Autodesk Inventor part; units mm, degrees
(part 8 of 12)
  line L6268 (-29.2354, 17.1217) -> (-29.7413, 17.6276)
  line L6269 (-29.7413, 17.6276) -> (-30.4567, 17.6276)
  line L6270 (-30.4567, 17.6276) -> (-30.9626, 17.1217)
  line L6271 (-30.9626, 17.1217) -> (-30.9626, 16.4063)
  line L6272 (-30.9626, 16.4063) -> (-30.4567, 15.9004)
  line L6273 (-30.4567, 15.9004) -> (-29.7413, 15.9004)
  line L6274 (-29.7413, 15.9004) -> (-29.2354, 16.4063)
  circle A475 centre (-30.099, 16.764) radius 0.8636
  circle A476 centre (-30.099, 16.764) radius 0.8636
  line L6275 (-29.2354, 16.4063) -> (-29.2354, 17.1217)
  line L6276 (-29.2354, 17.1217) -> (-29.7413, 17.6276)
  line L6277 (-29.7413, 17.6276) -> (-30.4567, 17.6276)
  line L6278 (-30.4567, 17.6276) -> (-30.9626, 17.1217)
  line L6279 (-30.9626, 17.1217) -> (-30.9626, 16.4063)
  line L6280 (-30.9626, 16.4063) -> (-30.4567, 15.9004)
  line L6281 (-30.4567, 15.9004) -> (-29.7413, 15.9004)
  line L6282 (-29.7413, 15.9004) -> (-29.2354, 16.4063)
  line L6283 (-29.2354, 13.8663) -> (-29.2354, 14.5817)
  line L6284 (-29.2354, 14.5817) -> (-29.7413, 15.0876)
  line L6285 (-29.7413, 15.0876) -> (-30.4567, 15.0876)
  line L6286 (-30.4567, 15.0876) -> (-30.9626, 14.5817)
  line L6287 (-30.9626, 14.5817) -> (-30.9626, 13.8663)
  line L6288 (-30.9626, 13.8663) -> (-30.4567, 13.3604)
  line L6289 (-30.4567, 13.3604) -> (-29.7413, 13.3604)
  line L6290 (-29.7413, 13.3604) -> (-29.2354, 13.8663)
  circle A477 centre (-30.099, 14.224) radius 0.8636
  circle A478 centre (-30.099, 14.224) radius 0.8636
  line L6291 (-29.2354, 13.8663) -> (-29.2354, 14.5817)
  line L6292 (-29.2354, 14.5817) -> (-29.7413, 15.0876)
  line L6293 (-29.7413, 15.0876) -> (-30.4567, 15.0876)
  line L6294 (-30.4567, 15.0876) -> (-30.9626, 14.5817)
  line L6295 (-30.9626, 14.5817) -> (-30.9626, 13.8663)
  line L6296 (-30.9626, 13.8663) -> (-30.4567, 13.3604)
  line L6297 (-30.4567, 13.3604) -> (-29.7413, 13.3604)
  line L6298 (-29.7413, 13.3604) -> (-29.2354, 13.8663)
  line L6299 (-29.2354, 11.3263) -> (-29.2354, 12.0417)
  line L6300 (-29.2354, 12.0417) -> (-29.7413, 12.5476)
  line L6301 (-29.7413, 12.5476) -> (-30.4567, 12.5476)
  line L6302 (-30.4567, 12.5476) -> (-30.9626, 12.0417)
  line L6303 (-30.9626, 12.0417) -> (-30.9626, 11.3263)
  line L6304 (-30.9626, 11.3263) -> (-30.4567, 10.8204)
  line L6305 (-30.4567, 10.8204) -> (-29.7413, 10.8204)
  line L6306 (-29.7413, 10.8204) -> (-29.2354, 11.3263)
  circle A479 centre (-30.099, 11.684) radius 0.8636
  circle A480 centre (-30.099, 11.684) radius 0.8636
  line L6307 (-29.2354, 11.3263) -> (-29.2354, 12.0417)
  line L6308 (-29.2354, 12.0417) -> (-29.7413, 12.5476)
  line L6309 (-29.7413, 12.5476) -> (-30.4567, 12.5476)
  line L6310 (-30.4567, 12.5476) -> (-30.9626, 12.0417)
  line L6311 (-30.9626, 12.0417) -> (-30.9626, 11.3263)
  line L6312 (-30.9626, 11.3263) -> (-30.4567, 10.8204)
  line L6313 (-30.4567, 10.8204) -> (-29.7413, 10.8204)
  line L6314 (-29.7413, 10.8204) -> (-29.2354, 11.3263)
  line L6315 (-29.2354, 8.7863) -> (-29.2354, 9.5017)
  line L6316 (-29.2354, 9.5017) -> (-29.7413, 10.0076)
  line L6317 (-29.7413, 10.0076) -> (-30.4567, 10.0076)
  line L6318 (-30.4567, 10.0076) -> (-30.9626, 9.5017)
  line L6319 (-30.9626, 9.5017) -> (-30.9626, 8.7863)
  line L6320 (-30.9626, 8.7863) -> (-30.4567, 8.2804)
  line L6321 (-30.4567, 8.2804) -> (-29.7413, 8.2804)
  line L6322 (-29.7413, 8.2804) -> (-29.2354, 8.7863)
  circle A481 centre (-30.099, 9.144) radius 0.8636
  circle A482 centre (-30.099, 9.144) radius 0.8636
  line L6323 (-29.2354, 8.7863) -> (-29.2354, 9.5017)
  line L6324 (-29.2354, 9.5017) -> (-29.7413, 10.0076)
  line L6325 (-29.7413, 10.0076) -> (-30.4567, 10.0076)
  line L6326 (-30.4567, 10.0076) -> (-30.9626, 9.5017)
  line L6327 (-30.9626, 9.5017) -> (-30.9626, 8.7863)
  line L6328 (-30.9626, 8.7863) -> (-30.4567, 8.2804)
  line L6329 (-30.4567, 8.2804) -> (-29.7413, 8.2804)
  line L6330 (-29.7413, 8.2804) -> (-29.2354, 8.7863)
  line L6331 (-29.2354, 6.2463) -> (-29.2354, 6.9617)
  line L6332 (-29.2354, 6.9617) -> (-29.7413, 7.4676)
  line L6333 (-29.7413, 7.4676) -> (-30.4567, 7.4676)
  line L6334 (-30.4567, 7.4676) -> (-30.9626, 6.9617)
  line L6335 (-30.9626, 6.9617) -> (-30.9626, 6.2463)
  line L6336 (-30.9626, 6.2463) -> (-30.4567, 5.7404)
  line L6337 (-30.4567, 5.7404) -> (-29.7413, 5.7404)
  line L6338 (-29.7413, 5.7404) -> (-29.2354, 6.2463)
  circle A483 centre (-30.099, 6.604) radius 0.8636
  circle A484 centre (-30.099, 6.604) radius 0.8636
  line L6339 (-29.2354, 6.2463) -> (-29.2354, 6.9617)
  line L6340 (-29.2354, 6.9617) -> (-29.7413, 7.4676)
  line L6341 (-29.7413, 7.4676) -> (-30.4567, 7.4676)
  line L6342 (-30.4567, 7.4676) -> (-30.9626, 6.9617)
  line L6343 (-30.9626, 6.9617) -> (-30.9626, 6.2463)
  line L6344 (-30.9626, 6.2463) -> (-30.4567, 5.7404)
  line L6345 (-30.4567, 5.7404) -> (-29.7413, 5.7404)
  line L6346 (-29.7413, 5.7404) -> (-29.2354, 6.2463)
  line L6347 (-4.453, 11.714) -> (-4.453, 10.714)
  line L6348 (-4.453, 10.714) -> (-5.453, 10.714)
  line L6349 (-5.453, 10.714) -> (-5.453, 11.714)
  line L6350 (-5.453, 11.714) -> (-4.453, 11.714)
  line L6351 (-4.453, 10.114) -> (-4.453, 9.114)
  line L6352 (-4.453, 9.114) -> (-5.453, 9.114)
  line L6353 (-5.453, 9.114) -> (-5.453, 10.114)
  line L6354 (-5.453, 10.114) -> (-4.453, 10.114)
  line L6355 (-24.287, 6.977) -> (-23.287, 6.977)
  line L6356 (-23.287, 6.977) -> (-23.287, 5.977)
  line L6357 (-23.287, 5.977) -> (-24.287, 5.977)
  line L6358 (-24.287, 5.977) -> (-24.287, 6.977)
  line L6359 (-22.687, 6.977) -> (-21.687, 6.977)
  line L6360 (-21.687, 6.977) -> (-21.687, 5.977)
  line L6361 (-21.687, 5.977) -> (-22.687, 5.977)
  line L6362 (-22.687, 5.977) -> (-22.687, 6.977)
  line L6363 (-2.74, 31.099) -> (-3.74, 31.099)
  line L6364 (-3.74, 31.099) -> (-3.74, 32.099)
  line L6365 (-3.74, 32.099) -> (-2.74, 32.099)
  line L6366 (-2.74, 32.099) -> (-2.74, 31.099)
  line L6367 (-2.74, 28.099) -> (-3.74, 28.099)
  line L6368 (-3.74, 28.099) -> (-3.74, 29.099)
  line L6369 (-3.74, 29.099) -> (-2.74, 29.099)
  line L6370 (-2.74, 29.099) -> (-2.74, 28.099)
  line L6371 (-1.34, 28.099) -> (-2.34, 28.099)
  line L6372 (-2.34, 28.099) -> (-2.34, 29.099)
  line L6373 (-2.34, 29.099) -> (-1.34, 29.099)
  line L6374 (-1.34, 29.099) -> (-1.34, 28.099)
  line L6375 (-1.34, 31.099) -> (-2.34, 31.099)
  line L6376 (-2.34, 31.099) -> (-2.34, 32.099)
  line L6377 (-2.34, 32.099) -> (-1.34, 32.099)
  line L6378 (-1.34, 32.099) -> (-1.34, 31.099)
  line L6379 (-34.8585, 34.5556) -> (-34.1514, 35.2627)
  line L6380 (-34.1514, 35.2627) -> (-33.4443, 34.5556)
  line L6381 (-33.4443, 34.5556) -> (-34.1514, 33.8485)
  line L6382 (-34.1514, 33.8485) -> (-34.8585, 34.5556)
  line L6383 (-32.5957, 36.8184) -> (-31.8886, 37.5255)
  line L6384 (-31.8886, 37.5255) -> (-31.1815, 36.8184)
  line L6385 (-31.1815, 36.8184) -> (-31.8886, 36.1113)
  line L6386 (-31.8886, 36.1113) -> (-32.5957, 36.8184)
  line L6387 (-3.6714, 37.5255) -> (-2.9643, 36.8184)
  line L6388 (-2.9643, 36.8184) -> (-3.6714, 36.1113)
  line L6389 (-3.6714, 36.1113) -> (-4.3785, 36.8184)
  line L6390 (-4.3785, 36.8184) -> (-3.6714, 37.5255)
  line L6391 (-1.4086, 35.2627) -> (-0.7015, 34.5556)
  line L6392 (-0.7015, 34.5556) -> (-1.4086, 33.8485)
  line L6393 (-1.4086, 33.8485) -> (-2.1157, 34.5556)
  line L6394 (-2.1157, 34.5556) -> (-1.4086, 35.2627)
  circle A485 centre (-7.78, 36.068) radius 2.2225
  circle A486 centre (-7.78, 36.068) radius 1.778
  circle A487 centre (-7.78, 36.068) radius 1.778
  circle A488 centre (-7.78, 36.068) radius 2.2225
  circle A489 centre (-27.78, 36.068) radius 2.2225
  circle A490 centre (-27.78, 36.068) radius 1.778
  circle A491 centre (-27.78, 36.068) radius 1.778
  circle A492 centre (-27.78, 36.068) radius 2.2225
  line L6395 (-2.106, 23.519) -> (-3.106, 23.519)
  line L6396 (-3.106, 23.519) -> (-3.106, 24.519)
  line L6397 (-3.106, 24.519) -> (-2.106, 24.519)
  line L6398 (-2.106, 24.519) -> (-2.106, 23.519)
  line L6399 (-4.006, 23.519) -> (-5.006, 23.519)
  line L6400 (-5.006, 23.519) -> (-5.006, 24.519)
  line L6401 (-5.006, 24.519) -> (-4.006, 24.519)
  line L6402 (-4.006, 24.519) -> (-4.006, 23.519)
  line L6403 (-3.056, 25.619) -> (-4.056, 25.619)
  line L6404 (-4.056, 25.619) -> (-4.056, 26.619)
  line L6405 (-4.056, 26.619) -> (-3.056, 26.619)
  line L6406 (-3.056, 26.619) -> (-3.056, 25.619)
  line L6407 (-5.469, 25.519) -> (-5.469, 24.519)
  line L6408 (-5.469, 24.519) -> (-6.469, 24.519)
  line L6409 (-6.469, 24.519) -> (-6.469, 25.519)
  line L6410 (-6.469, 25.519) -> (-5.469, 25.519)
  line L6411 (-5.469, 26.369) -> (-5.469, 25.369)
  line L6412 (-5.469, 25.369) -> (-6.469, 25.369)
  line L6413 (-6.469, 25.369) -> (-6.469, 26.369)
  line L6414 (-6.469, 26.369) -> (-5.469, 26.369)
  line L6415 (-5.469, 24.669) -> (-5.469, 23.669)
  line L6416 (-5.469, 23.669) -> (-6.469, 23.669)
  line L6417 (-6.469, 23.669) -> (-6.469, 24.669)
  line L6418 (-6.469, 24.669) -> (-5.469, 24.669)
  line L6419 (-0.643, 25.519) -> (-0.643, 24.519)
  line L6420 (-0.643, 24.519) -> (-1.643, 24.519)
  line L6421 (-1.643, 24.519) -> (-1.643, 25.519)
  line L6422 (-1.643, 25.519) -> (-0.643, 25.519)
  line L6423 (-0.643, 26.369) -> (-0.643, 25.369)
  line L6424 (-0.643, 25.369) -> (-1.643, 25.369)
  line L6425 (-1.643, 25.369) -> (-1.643, 26.369)
  line L6426 (-1.643, 26.369) -> (-0.643, 26.369)
  line L6427 (-0.643, 24.669) -> (-0.643, 23.669)
  line L6428 (-0.643, 23.669) -> (-1.643, 23.669)
  line L6429 (-1.643, 23.669) -> (-1.643, 24.669)
  line L6430 (-1.643, 24.669) -> (-0.643, 24.669)
  line L6431 (-19.804, 30.599) -> (-18.804, 30.599)
  line L6432 (-18.804, 30.599) -> (-18.804, 29.599)
  line L6433 (-18.804, 29.599) -> (-19.804, 29.599)
  line L6434 (-19.804, 29.599) -> (-19.804, 30.599)
  line L6435 (-20.654, 30.599) -> (-19.654, 30.599)
  line L6436 (-19.654, 30.599) -> (-19.654, 29.599)
  line L6437 (-19.654, 29.599) -> (-20.654, 29.599)
  line L6438 (-20.654, 29.599) -> (-20.654, 30.599)
  line L6439 (-18.954, 30.599) -> (-17.954, 30.599)
  line L6440 (-17.954, 30.599) -> (-17.954, 29.599)
  line L6441 (-17.954, 29.599) -> (-18.954, 29.599)
  line L6442 (-18.954, 29.599) -> (-18.954, 30.599)
  line L6443 (-23.2, 32.7) -> (-23.2, 31.7)
  line L6444 (-23.2, 31.7) -> (-24.2, 31.7)
  line L6445 (-24.2, 31.7) -> (-24.2, 32.7)
  line L6446 (-24.2, 32.7) -> (-23.2, 32.7)
  line L6447 (-23.2, 33.55) -> (-23.2, 32.55)
  line L6448 (-23.2, 32.55) -> (-24.2, 32.55)
  line L6449 (-24.2, 32.55) -> (-24.2, 33.55)
  line L6450 (-24.2, 33.55) -> (-23.2, 33.55)
  line L6451 (-23.2, 31.85) -> (-23.2, 30.85)
  line L6452 (-23.2, 30.85) -> (-24.2, 30.85)
  line L6453 (-24.2, 30.85) -> (-24.2, 31.85)
  line L6454 (-24.2, 31.85) -> (-23.2, 31.85)
  line L6455 (-5.1385, 32.053) -> (-5.1385, 31.053)
  line L6456 (-5.1385, 31.053) -> (-6.1385, 31.053)
  line L6457 (-6.1385, 31.053) -> (-6.1385, 32.053)
  line L6458 (-6.1385, 32.053) -> (-5.1385, 32.053)
  line L6459 (-5.1385, 31.253) -> (-5.1385, 30.253)
  line L6460 (-5.1385, 30.253) -> (-6.1385, 30.253)
  line L6461 (-6.1385, 30.253) -> (-6.1385, 31.253)
  line L6462 (-6.1385, 31.253) -> (-5.1385, 31.253)
  line L6463 (-5.1385, 30.453) -> (-5.1385, 29.453)
  line L6464 (-5.1385, 29.453) -> (-6.1385, 29.453)
  line L6465 (-6.1385, 29.453) -> (-6.1385, 30.453)
  line L6466 (-6.1385, 30.453) -> (-5.1385, 30.453)
  line L6467 (-5.1385, 29.653) -> (-5.1385, 28.653)
  line L6468 (-5.1385, 28.653) -> (-6.1385, 28.653)
  line L6469 (-6.1385, 28.653) -> (-6.1385, 29.653)
  line L6470 (-6.1385, 29.653) -> (-5.1385, 29.653)
  line L6471 (-7.6885, 28.653) -> (-7.6885, 29.653)
  line L6472 (-7.6885, 29.653) -> (-6.6885, 29.653)
  line L6473 (-6.6885, 29.653) -> (-6.6885, 28.653)
  line L6474 (-6.6885, 28.653) -> (-7.6885, 28.653)
  line L6475 (-7.6885, 29.453) -> (-7.6885, 30.453)
  line L6476 (-7.6885, 30.453) -> (-6.6885, 30.453)
  line L6477 (-6.6885, 30.453) -> (-6.6885, 29.453)
  line L6478 (-6.6885, 29.453) -> (-7.6885, 29.453)
  line L6479 (-7.6885, 30.253) -> (-7.6885, 31.253)
  line L6480 (-7.6885, 31.253) -> (-6.6885, 31.253)
  line L6481 (-6.6885, 31.253) -> (-6.6885, 30.253)
  line L6482 (-6.6885, 30.253) -> (-7.6885, 30.253)
  line L6483 (-7.6885, 31.053) -> (-7.6885, 32.053)
  line L6484 (-7.6885, 32.053) -> (-6.6885, 32.053)
  line L6485 (-6.6885, 32.053) -> (-6.6885, 31.053)
  line L6486 (-6.6885, 31.053) -> (-7.6885, 31.053)
  line L6487 (-26.792, 24.941) -> (-26.792, 23.941)
  line L6488 (-26.792, 23.941) -> (-27.792, 23.941)
  line L6489 (-27.792, 23.941) -> (-27.792, 24.941)
  line L6490 (-27.792, 24.941) -> (-26.792, 24.941)
  line L6491 (-26.792, 24.141) -> (-26.792, 23.141)
  line L6492 (-26.792, 23.141) -> (-27.792, 23.141)
  line L6493 (-27.792, 23.141) -> (-27.792, 24.141)
  line L6494 (-27.792, 24.141) -> (-26.792, 24.141)
  line L6495 (-26.792, 23.341) -> (-26.792, 22.341)
  line L6496 (-26.792, 22.341) -> (-27.792, 22.341)
  line L6497 (-27.792, 22.341) -> (-27.792, 23.341)
  line L6498 (-27.792, 23.341) -> (-26.792, 23.341)
  line L6499 (-26.792, 22.541) -> (-26.792, 21.541)
  line L6500 (-26.792, 21.541) -> (-27.792, 21.541)
  line L6501 (-27.792, 21.541) -> (-27.792, 22.541)
  line L6502 (-27.792, 22.541) -> (-26.792, 22.541)
  line L6503 (-29.342, 21.541) -> (-29.342, 22.541)
  line L6504 (-29.342, 22.541) -> (-28.342, 22.541)
  line L6505 (-28.342, 22.541) -> (-28.342, 21.541)
  line L6506 (-28.342, 21.541) -> (-29.342, 21.541)
  line L6507 (-29.342, 22.341) -> (-29.342, 23.341)
  line L6508 (-29.342, 23.341) -> (-28.342, 23.341)
  line L6509 (-28.342, 23.341) -> (-28.342, 22.341)
  line L6510 (-28.342, 22.341) -> (-29.342, 22.341)
  line L6511 (-29.342, 23.141) -> (-29.342, 24.141)
  line L6512 (-29.342, 24.141) -> (-28.342, 24.141)
  line L6513 (-28.342, 24.141) -> (-28.342, 23.141)
  line L6514 (-28.342, 23.141) -> (-29.342, 23.141)
  line L6515 (-29.342, 23.941) -> (-29.342, 24.941)
  line L6516 (-29.342, 24.941) -> (-28.342, 24.941)
  line L6517 (-28.342, 24.941) -> (-28.342, 23.941)
  line L6518 (-28.342, 23.941) -> (-29.342, 23.941)
  line L6519 (-26.792, 32.434) -> (-26.792, 31.434)
  line L6520 (-26.792, 31.434) -> (-27.792, 31.434)
  line L6521 (-27.792, 31.434) -> (-27.792, 32.434)
  line L6522 (-27.792, 32.434) -> (-26.792, 32.434)
  line L6523 (-26.792, 31.634) -> (-26.792, 30.634)
  line L6524 (-26.792, 30.634) -> (-27.792, 30.634)
  line L6525 (-27.792, 30.634) -> (-27.792, 31.634)
  line L6526 (-27.792, 31.634) -> (-26.792, 31.634)
  line L6527 (-26.792, 30.834) -> (-26.792, 29.834)
  line L6528 (-26.792, 29.834) -> (-27.792, 29.834)
  line L6529 (-27.792, 29.834) -> (-27.792, 30.834)
  line L6530 (-27.792, 30.834) -> (-26.792, 30.834)
  line L6531 (-26.792, 30.034) -> (-26.792, 29.034)
  line L6532 (-26.792, 29.034) -> (-27.792, 29.034)
  line L6533 (-27.792, 29.034) -> (-27.792, 30.034)
  line L6534 (-27.792, 30.034) -> (-26.792, 30.034)
  line L6535 (-29.342, 29.034) -> (-29.342, 30.034)
  line L6536 (-29.342, 30.034) -> (-28.342, 30.034)
  line L6537 (-28.342, 30.034) -> (-28.342, 29.034)
  line L6538 (-28.342, 29.034) -> (-29.342, 29.034)
  line L6539 (-29.342, 29.834) -> (-29.342, 30.834)
  line L6540 (-29.342, 30.834) -> (-28.342, 30.834)
  line L6541 (-28.342, 30.834) -> (-28.342, 29.834)
  line L6542 (-28.342, 29.834) -> (-29.342, 29.834)
  line L6543 (-29.342, 30.634) -> (-29.342, 31.634)
  line L6544 (-29.342, 31.634) -> (-28.342, 31.634)
  line L6545 (-28.342, 31.634) -> (-28.342, 30.634)
  line L6546 (-28.342, 30.634) -> (-29.342, 30.634)
  line L6547 (-29.342, 31.434) -> (-29.342, 32.434)
  line L6548 (-29.342, 32.434) -> (-28.342, 32.434)
  line L6549 (-28.342, 32.434) -> (-28.342, 31.434)
  line L6550 (-28.342, 31.434) -> (-29.342, 31.434)
  line L6551 (-13.7, 30.325) -> (-14.7, 30.325)
  line L6552 (-14.7, 30.325) -> (-14.7, 31.325)
  line L6553 (-14.7, 31.325) -> (-13.7, 31.325)
  line L6554 (-13.7, 31.325) -> (-13.7, 30.325)
  line L6555 (-14.5, 30.325) -> (-15.5, 30.325)
  line L6556 (-15.5, 30.325) -> (-15.5, 31.325)
  line L6557 (-15.5, 31.325) -> (-14.5, 31.325)
  line L6558 (-14.5, 31.325) -> (-14.5, 30.325)
  line L6559 (-15.5, 32.875) -> (-14.5, 32.875)
  line L6560 (-14.5, 32.875) -> (-14.5, 31.875)
  line L6561 (-14.5, 31.875) -> (-15.5, 31.875)
  line L6562 (-15.5, 31.875) -> (-15.5, 32.875)
  line L6563 (-14.7, 32.875) -> (-13.7, 32.875)
  line L6564 (-13.7, 32.875) -> (-13.7, 31.875)
  line L6565 (-13.7, 31.875) -> (-14.7, 31.875)
  line L6566 (-14.7, 31.875) -> (-14.7, 32.875)
  line L6567 (-13.7367, 24.3158) -> (-14.7367, 24.3158)
  line L6568 (-14.7367, 24.3158) -> (-14.7367, 25.3158)
  line L6569 (-14.7367, 25.3158) -> (-13.7367, 25.3158)
  line L6570 (-13.7367, 25.3158) -> (-13.7367, 24.3158)
  line L6571 (-15.4512, 24.3158) -> (-16.4512, 24.3158)
  line L6572 (-16.4512, 24.3158) -> (-16.4512, 25.3158)
  line L6573 (-16.4512, 25.3158) -> (-15.4512, 25.3158)
  line L6574 (-15.4512, 25.3158) -> (-15.4512, 24.3158)
  line L6575 (-13.7367, 24.3412) -> (-14.7367, 24.3412)
  line L6576 (-14.7367, 24.3412) -> (-14.7367, 25.3412)
  line L6577 (-14.7367, 25.3412) -> (-13.7367, 25.3412)
  line L6578 (-13.7367, 25.3412) -> (-13.7367, 24.3412)
  line L6579 (-15.4512, 24.3412) -> (-16.4512, 24.3412)
  line L6580 (-16.4512, 24.3412) -> (-16.4512, 25.3412)
  line L6581 (-16.4512, 25.3412) -> (-15.4512, 25.3412)
  line L6582 (-15.4512, 25.3412) -> (-15.4512, 24.3412)
  line L6583 (-13.7748, 24.3666) -> (-14.7748, 24.3666)
  line L6584 (-14.7748, 24.3666) -> (-14.7748, 25.3666)
  line L6585 (-14.7748, 25.3666) -> (-13.7748, 25.3666)
  line L6586 (-13.7748, 25.3666) -> (-13.7748, 24.3666)
  line L6587 (-15.4512, 24.3666) -> (-16.4512, 24.3666)
  line L6588 (-16.4512, 24.3666) -> (-16.4512, 25.3666)
  line L6589 (-16.4512, 25.3666) -> (-15.4512, 25.3666)
  line L6590 (-15.4512, 25.3666) -> (-15.4512, 24.3666)
  line L6591 (-13.8256, 24.392) -> (-14.8256, 24.392)
  line L6592 (-14.8256, 24.392) -> (-14.8256, 25.392)
  line L6593 (-14.8256, 25.392) -> (-13.8256, 25.392)
  line L6594 (-13.8256, 25.392) -> (-13.8256, 24.392)
  line L6595 (-15.4512, 24.392) -> (-16.4512, 24.392)
  line L6596 (-16.4512, 24.392) -> (-16.4512, 25.392)
  line L6597 (-16.4512, 25.392) -> (-15.4512, 25.392)
  line L6598 (-15.4512, 25.392) -> (-15.4512, 24.392)
  line L6599 (-13.7287, 24.9047) -> (-13.7541, 24.9047)
  line L6600 (-13.7541, 24.9047) -> (-13.7541, 24.9301)
  line L6601 (-13.7541, 24.9301) -> (-13.7287, 24.9301)
  line L6602 (-13.7287, 24.9301) -> (-13.7287, 24.9047)
  line L6603 (-13.851, 24.4174) -> (-14.851, 24.4174)
  line L6604 (-14.851, 24.4174) -> (-14.851, 25.4174)
  line L6605 (-14.851, 25.4174) -> (-13.851, 25.4174)
  line L6606 (-13.851, 25.4174) -> (-13.851, 24.4174)
  line L6607 (-15.4512, 24.4174) -> (-16.4512, 24.4174)
  line L6608 (-16.4512, 24.4174) -> (-16.4512, 25.4174)
  line L6609 (-16.4512, 25.4174) -> (-15.4512, 25.4174)
  line L6610 (-15.4512, 25.4174) -> (-15.4512, 24.4174)
  line L6611 (-13.216, 24.4428) -> (-14.216, 24.4428)
  line L6612 (-14.216, 24.4428) -> (-14.216, 25.4428)
  line L6613 (-14.216, 25.4428) -> (-13.216, 25.4428)
  line L6614 (-13.216, 25.4428) -> (-13.216, 24.4428)
  line L6615 (-13.8764, 24.4428) -> (-14.8764, 24.4428)
  line L6616 (-14.8764, 24.4428) -> (-14.8764, 25.4428)
  line L6617 (-14.8764, 25.4428) -> (-13.8764, 25.4428)
  line L6618 (-13.8764, 25.4428) -> (-13.8764, 24.4428)
  line L6619 (-15.4512, 24.4428) -> (-16.4512, 24.4428)
  line L6620 (-16.4512, 24.4428) -> (-16.4512, 25.4428)
  line L6621 (-16.4512, 25.4428) -> (-15.4512, 25.4428)
  line L6622 (-15.4512, 25.4428) -> (-15.4512, 24.4428)
  line L6623 (-13.1906, 24.4682) -> (-14.1906, 24.4682)
  line L6624 (-14.1906, 24.4682) -> (-14.1906, 25.4682)
  line L6625 (-14.1906, 25.4682) -> (-13.1906, 25.4682)
  line L6626 (-13.1906, 25.4682) -> (-13.1906, 24.4682)
  line L6627 (-13.9018, 24.4682) -> (-14.9018, 24.4682)
  line L6628 (-14.9018, 24.4682) -> (-14.9018, 25.4682)
  line L6629 (-14.9018, 25.4682) -> (-13.9018, 25.4682)
  line L6630 (-13.9018, 25.4682) -> (-13.9018, 24.4682)
  line L6631 (-15.4639, 24.4682) -> (-16.4639, 24.4682)
  line L6632 (-16.4639, 24.4682) -> (-16.4639, 25.4682)
  line L6633 (-16.4639, 25.4682) -> (-15.4639, 25.4682)
  line L6634 (-15.4639, 25.4682) -> (-15.4639, 24.4682)
  line L6635 (-13.1652, 24.4936) -> (-14.1652, 24.4936)
  line L6636 (-14.1652, 24.4936) -> (-14.1652, 25.4936)
  line L6637 (-14.1652, 25.4936) -> (-13.1652, 25.4936)
  line L6638 (-13.1652, 25.4936) -> (-13.1652, 24.4936)
  line L6639 (-13.9272, 24.4936) -> (-14.9272, 24.4936)
  line L6640 (-14.9272, 24.4936) -> (-14.9272, 25.4936)
  line L6641 (-14.9272, 25.4936) -> (-13.9272, 25.4936)
  line L6642 (-13.9272, 25.4936) -> (-13.9272, 24.4936)
  line L6643 (-15.4639, 24.4936) -> (-16.4639, 24.4936)
  line L6644 (-16.4639, 24.4936) -> (-16.4639, 25.4936)
  line L6645 (-16.4639, 25.4936) -> (-15.4639, 25.4936)
  line L6646 (-15.4639, 25.4936) -> (-15.4639, 24.4936)
  line L6647 (-13.1525, 24.519) -> (-14.1525, 24.519)
  line L6648 (-14.1525, 24.519) -> (-14.1525, 25.519)
  line L6649 (-14.1525, 25.519) -> (-13.1525, 25.519)
  line L6650 (-13.1525, 25.519) -> (-13.1525, 24.519)
  line L6651 (-13.9526, 24.519) -> (-14.9526, 24.519)
  line L6652 (-14.9526, 24.519) -> (-14.9526, 25.519)
  line L6653 (-14.9526, 25.519) -> (-13.9526, 25.519)
  line L6654 (-13.9526, 25.519) -> (-13.9526, 24.519)
  line L6655 (-15.4639, 24.519) -> (-16.4639, 24.519)
  line L6656 (-16.4639, 24.519) -> (-16.4639, 25.519)
  line L6657 (-16.4639, 25.519) -> (-15.4639, 25.519)
  line L6658 (-15.4639, 25.519) -> (-15.4639, 24.519)
  line L6659 (-13.1271, 24.5444) -> (-14.1271, 24.5444)
  line L6660 (-14.1271, 24.5444) -> (-14.1271, 25.5444)
  line L6661 (-14.1271, 25.5444) -> (-13.1271, 25.5444)
  line L6662 (-13.1271, 25.5444) -> (-13.1271, 24.5444)
  line L6663 (-13.9653, 24.5444) -> (-14.9653, 24.5444)
  line L6664 (-14.9653, 24.5444) -> (-14.9653, 25.5444)
  line L6665 (-14.9653, 25.5444) -> (-13.9653, 25.5444)
  line L6666 (-13.9653, 25.5444) -> (-13.9653, 24.5444)
  line L6667 (-15.4639, 24.5444) -> (-16.4639, 24.5444)
  line L6668 (-16.4639, 24.5444) -> (-16.4639, 25.5444)
  line L6669 (-16.4639, 25.5444) -> (-15.4639, 25.5444)
  line L6670 (-15.4639, 25.5444) -> (-15.4639, 24.5444)
  line L6671 (-13.1144, 24.5698) -> (-14.1144, 24.5698)
  line L6672 (-14.1144, 24.5698) -> (-14.1144, 25.5698)
  line L6673 (-14.1144, 25.5698) -> (-13.1144, 25.5698)
  line L6674 (-13.1144, 25.5698) -> (-13.1144, 24.5698)
  line L6675 (-13.9907, 24.5698) -> (-14.9907, 24.5698)
  line L6676 (-14.9907, 24.5698) -> (-14.9907, 25.5698)
  line L6677 (-14.9907, 25.5698) -> (-13.9907, 25.5698)
  line L6678 (-13.9907, 25.5698) -> (-13.9907, 24.5698)
  line L6679 (-15.4639, 24.5698) -> (-16.4639, 24.5698)
  line L6680 (-16.4639, 24.5698) -> (-16.4639, 25.5698)
  line L6681 (-16.4639, 25.5698) -> (-15.4639, 25.5698)
  line L6682 (-15.4639, 25.5698) -> (-15.4639, 24.5698)
  line L6683 (-13.1017, 24.5952) -> (-14.1017, 24.5952)
  line L6684 (-14.1017, 24.5952) -> (-14.1017, 25.5952)
  line L6685 (-14.1017, 25.5952) -> (-13.1017, 25.5952)
  line L6686 (-13.1017, 25.5952) -> (-13.1017, 24.5952)
  line L6687 (-14.0034, 24.5952) -> (-15.0034, 24.5952)
  line L6688 (-15.0034, 24.5952) -> (-15.0034, 25.5952)
  line L6689 (-15.0034, 25.5952) -> (-14.0034, 25.5952)
  line L6690 (-14.0034, 25.5952) -> (-14.0034, 24.5952)
  line L6691 (-15.4639, 24.5952) -> (-16.4639, 24.5952)
  line L6692 (-16.4639, 24.5952) -> (-16.4639, 25.5952)
  line L6693 (-16.4639, 25.5952) -> (-15.4639, 25.5952)
  line L6694 (-15.4639, 25.5952) -> (-15.4639, 24.5952)
  line L6695 (-13.0763, 24.6206) -> (-14.0763, 24.6206)
  line L6696 (-14.0763, 24.6206) -> (-14.0763, 25.6206)
  line L6697 (-14.0763, 25.6206) -> (-13.0763, 25.6206)
  line L6698 (-13.0763, 25.6206) -> (-13.0763, 24.6206)
  line L6699 (-13.978, 24.6206) -> (-14.978, 24.6206)
  line L6700 (-14.978, 24.6206) -> (-14.978, 25.6206)
  line L6701 (-14.978, 25.6206) -> (-13.978, 25.6206)
  line L6702 (-13.978, 25.6206) -> (-13.978, 24.6206)
  line L6703 (-15.4639, 24.6206) -> (-16.4639, 24.6206)
  line L6704 (-16.4639, 24.6206) -> (-16.4639, 25.6206)
  line L6705 (-16.4639, 25.6206) -> (-15.4639, 25.6206)
  line L6706 (-15.4639, 25.6206) -> (-15.4639, 24.6206)
  line L6707 (-13.0636, 24.646) -> (-14.0636, 24.646)
  line L6708 (-14.0636, 24.646) -> (-14.0636, 25.646)
  line L6709 (-14.0636, 25.646) -> (-13.0636, 25.646)
  line L6710 (-13.0636, 25.646) -> (-13.0636, 24.646)
  line L6711 (-13.9526, 24.646) -> (-14.9526, 24.646)
  line L6712 (-14.9526, 24.646) -> (-14.9526, 25.646)
  line L6713 (-14.9526, 25.646) -> (-13.9526, 25.646)
  line L6714 (-13.9526, 25.646) -> (-13.9526, 24.646)
  line L6715 (-15.4639, 24.646) -> (-16.4639, 24.646)
  line L6716 (-16.4639, 24.646) -> (-16.4639, 25.646)
  line L6717 (-16.4639, 25.646) -> (-15.4639, 25.646)
  line L6718 (-15.4639, 25.646) -> (-15.4639, 24.646)
  line L6719 (-13.0509, 24.6714) -> (-14.0509, 24.6714)
  line L6720 (-14.0509, 24.6714) -> (-14.0509, 25.6714)
  line L6721 (-14.0509, 25.6714) -> (-13.0509, 25.6714)
  line L6722 (-13.0509, 25.6714) -> (-13.0509, 24.6714)
  line L6723 (-13.9272, 24.6714) -> (-14.9272, 24.6714)
  line L6724 (-14.9272, 24.6714) -> (-14.9272, 25.6714)
  line L6725 (-14.9272, 25.6714) -> (-13.9272, 25.6714)
  line L6726 (-13.9272, 25.6714) -> (-13.9272, 24.6714)
  line L6727 (-15.4766, 24.6714) -> (-16.4766, 24.6714)
  line L6728 (-16.4766, 24.6714) -> (-16.4766, 25.6714)
  line L6729 (-16.4766, 25.6714) -> (-15.4766, 25.6714)
  line L6730 (-15.4766, 25.6714) -> (-15.4766, 24.6714)
  line L6731 (-13.0382, 24.6968) -> (-14.0382, 24.6968)
  line L6732 (-14.0382, 24.6968) -> (-14.0382, 25.6968)
  line L6733 (-14.0382, 25.6968) -> (-13.0382, 25.6968)
  line L6734 (-13.0382, 25.6968) -> (-13.0382, 24.6968)
  line L6735 (-13.9145, 24.6968) -> (-14.9145, 24.6968)
  line L6736 (-14.9145, 24.6968) -> (-14.9145, 25.6968)
  line L6737 (-14.9145, 25.6968) -> (-13.9145, 25.6968)
  line L6738 (-13.9145, 25.6968) -> (-13.9145, 24.6968)
  line L6739 (-15.4766, 24.6968) -> (-16.4766, 24.6968)
  line L6740 (-16.4766, 24.6968) -> (-16.4766, 25.6968)
  line L6741 (-16.4766, 25.6968) -> (-15.4766, 25.6968)
  line L6742 (-15.4766, 25.6968) -> (-15.4766, 24.6968)
  line L6743 (-13.0255, 24.7222) -> (-14.0255, 24.7222)
  line L6744 (-14.0255, 24.7222) -> (-14.0255, 25.7222)
  line L6745 (-14.0255, 25.7222) -> (-13.0255, 25.7222)
  line L6746 (-13.0255, 25.7222) -> (-13.0255, 24.7222)
  line L6747 (-13.8891, 24.7222) -> (-14.8891, 24.7222)
  line L6748 (-14.8891, 24.7222) -> (-14.8891, 25.7222)
  line L6749 (-14.8891, 25.7222) -> (-13.8891, 25.7222)
  line L6750 (-13.8891, 25.7222) -> (-13.8891, 24.7222)
  line L6751 (-15.4766, 24.7222) -> (-16.4766, 24.7222)
  line L6752 (-16.4766, 24.7222) -> (-16.4766, 25.7222)
  line L6753 (-16.4766, 25.7222) -> (-15.4766, 25.7222)
  line L6754 (-15.4766, 25.7222) -> (-15.4766, 24.7222)
  line L6755 (-13.0128, 24.7476) -> (-14.0128, 24.7476)
  line L6756 (-14.0128, 24.7476) -> (-14.0128, 25.7476)
  line L6757 (-14.0128, 25.7476) -> (-13.0128, 25.7476)
  line L6758 (-13.0128, 25.7476) -> (-13.0128, 24.7476)
  line L6759 (-13.8637, 24.7476) -> (-14.8637, 24.7476)
  line L6760 (-14.8637, 24.7476) -> (-14.8637, 25.7476)
  line L6761 (-14.8637, 25.7476) -> (-13.8637, 25.7476)
  line L6762 (-13.8637, 25.7476) -> (-13.8637, 24.7476)
  line L6763 (-14.6892, 24.7476) -> (-15.6892, 24.7476)
  line L6764 (-15.6892, 24.7476) -> (-15.6892, 25.7476)
  line L6765 (-15.6892, 25.7476) -> (-14.6892, 25.7476)
  line L6766 (-14.6892, 25.7476) -> (-14.6892, 24.7476)
  line L6767 (-15.4766, 24.7476) -> (-16.4766, 24.7476)
  line L6768 (-16.4766, 24.7476) -> (-16.4766, 25.7476)
  line L6769 (-16.4766, 25.7476) -> (-15.4766, 25.7476)
  line L6770 (-15.4766, 25.7476) -> (-15.4766, 24.7476)
  line L6771 (-15.9973, 24.7476) -> (-16.9973, 24.7476)
  line L6772 (-16.9973, 24.7476) -> (-16.9973, 25.7476)
  line L6773 (-16.9973, 25.7476) -> (-15.9973, 25.7476)
  line L6774 (-15.9973, 25.7476) -> (-15.9973, 24.7476)
  line L6775 (-17.1403, 24.7476) -> (-18.1403, 24.7476)
  line L6776 (-18.1403, 24.7476) -> (-18.1403, 25.7476)
  line L6777 (-18.1403, 25.7476) -> (-17.1403, 25.7476)
  line L6778 (-17.1403, 25.7476) -> (-17.1403, 24.7476)
  line L6779 (-13.0001, 24.773) -> (-14.0001, 24.773)
  line L6780 (-14.0001, 24.773) -> (-14.0001, 25.773)
  line L6781 (-14.0001, 25.773) -> (-13.0001, 25.773)
  line L6782 (-13.0001, 25.773) -> (-13.0001, 24.773)
  line L6783 (-13.8383, 24.773) -> (-14.8383, 24.773)
  line L6784 (-14.8383, 24.773) -> (-14.8383, 25.773)
  line L6785 (-14.8383, 25.773) -> (-13.8383, 25.773)
  line L6786 (-13.8383, 25.773) -> (-13.8383, 24.773)
  line L6787 (-14.6765, 24.773) -> (-15.6765, 24.773)
  line L6788 (-15.6765, 24.773) -> (-15.6765, 25.773)
  line L6789 (-15.6765, 25.773) -> (-14.6765, 25.773)
  line L6790 (-14.6765, 25.773) -> (-14.6765, 24.773)
  line L6791 (-15.4766, 24.773) -> (-16.4766, 24.773)
  line L6792 (-16.4766, 24.773) -> (-16.4766, 25.773)
  line L6793 (-16.4766, 25.773) -> (-15.4766, 25.773)
  line L6794 (-15.4766, 25.773) -> (-15.4766, 24.773)
  line L6795 (-15.9973, 24.773) -> (-16.9973, 24.773)
  line L6796 (-16.9973, 24.773) -> (-16.9973, 25.773)
  line L6797 (-16.9973, 25.773) -> (-15.9973, 25.773)
  line L6798 (-15.9973, 25.773) -> (-15.9973, 24.773)
  line L6799 (-17.153, 24.773) -> (-18.153, 24.773)
  line L6800 (-18.153, 24.773) -> (-18.153, 25.773)
  line L6801 (-18.153, 25.773) -> (-17.153, 25.773)
  line L6802 (-17.153, 25.773) -> (-17.153, 24.773)
  line L6803 (-17.915, 24.773) -> (-18.915, 24.773)
  line L6804 (-18.915, 24.773) -> (-18.915, 25.773)
  line L6805 (-18.915, 25.773) -> (-17.915, 25.773)
  line L6806 (-17.915, 25.773) -> (-17.915, 24.773)
  line L6807 (-18.677, 24.773) -> (-19.677, 24.773)
  line L6808 (-19.677, 24.773) -> (-19.677, 25.773)
  line L6809 (-19.677, 25.773) -> (-18.677, 25.773)
  line L6810 (-18.677, 25.773) -> (-18.677, 24.773)
  line L6811 (-19.2358, 24.773) -> (-20.2358, 24.773)
  line L6812 (-20.2358, 24.773) -> (-20.2358, 25.773)
  line L6813 (-20.2358, 25.773) -> (-19.2358, 25.773)
  line L6814 (-19.2358, 25.773) -> (-19.2358, 24.773)
  line L6815 (-19.8327, 24.773) -> (-20.8327, 24.773)
  line L6816 (-20.8327, 24.773) -> (-20.8327, 25.773)
  line L6817 (-20.8327, 25.773) -> (-19.8327, 25.773)
  line L6818 (-19.8327, 25.773) -> (-19.8327, 24.773)
  line L6819 (-20.4677, 24.773) -> (-21.4677, 24.773)
  line L6820 (-21.4677, 24.773) -> (-21.4677, 25.773)
  line L6821 (-21.4677, 25.773) -> (-20.4677, 25.773)
  line L6822 (-20.4677, 25.773) -> (-20.4677, 24.773)
  line L6823 (-21.471, 24.773) -> (-22.471, 24.773)
  line L6824 (-22.471, 24.773) -> (-22.471, 25.773)
  line L6825 (-22.471, 25.773) -> (-21.471, 25.773)
  line L6826 (-21.471, 25.773) -> (-21.471, 24.773)
  line L6827 (-12.9874, 24.7984) -> (-13.9874, 24.7984)
  line L6828 (-13.9874, 24.7984) -> (-13.9874, 25.7984)
  line L6829 (-13.9874, 25.7984) -> (-12.9874, 25.7984)
  line L6830 (-12.9874, 25.7984) -> (-12.9874, 24.7984)
  line L6831 (-13.8256, 24.7984) -> (-14.8256, 24.7984)
  line L6832 (-14.8256, 24.7984) -> (-14.8256, 25.7984)
  line L6833 (-14.8256, 25.7984) -> (-13.8256, 25.7984)
  line L6834 (-13.8256, 25.7984) -> (-13.8256, 24.7984)
  line L6835 (-14.6765, 24.7984) -> (-15.6765, 24.7984)
  line L6836 (-15.6765, 24.7984) -> (-15.6765, 25.7984)
  line L6837 (-15.6765, 25.7984) -> (-14.6765, 25.7984)
  line L6838 (-14.6765, 25.7984) -> (-14.6765, 24.7984)
  line L6839 (-15.4766, 24.7984) -> (-16.4766, 24.7984)
  line L6840 (-16.4766, 24.7984) -> (-16.4766, 25.7984)
  line L6841 (-16.4766, 25.7984) -> (-15.4766, 25.7984)
  line L6842 (-15.4766, 25.7984) -> (-15.4766, 24.7984)
  line L6843 (-15.9846, 24.7984) -> (-16.9846, 24.7984)
  line L6844 (-16.9846, 24.7984) -> (-16.9846, 25.7984)
  line L6845 (-16.9846, 25.7984) -> (-15.9846, 25.7984)
  line L6846 (-15.9846, 25.7984) -> (-15.9846, 24.7984)
  line L6847 (-17.1276, 24.7984) -> (-18.1276, 24.7984)
  line L6848 (-18.1276, 24.7984) -> (-18.1276, 25.7984)
  line L6849 (-18.1276, 25.7984) -> (-17.1276, 25.7984)
  line L6850 (-17.1276, 25.7984) -> (-17.1276, 24.7984)
  line L6851 (-17.915, 24.7984) -> (-18.915, 24.7984)
  line L6852 (-18.915, 24.7984) -> (-18.915, 25.7984)
  line L6853 (-18.915, 25.7984) -> (-17.915, 25.7984)
  line L6854 (-17.915, 25.7984) -> (-17.915, 24.7984)
  line L6855 (-18.677, 24.7984) -> (-19.677, 24.7984)
  line L6856 (-19.677, 24.7984) -> (-19.677, 25.7984)
  line L6857 (-19.677, 25.7984) -> (-18.677, 25.7984)
  line L6858 (-18.677, 25.7984) -> (-18.677, 24.7984)
  line L6859 (-19.2358, 24.7984) -> (-20.2358, 24.7984)
  line L6860 (-20.2358, 24.7984) -> (-20.2358, 25.7984)
  line L6861 (-20.2358, 25.7984) -> (-19.2358, 25.7984)
  line L6862 (-19.2358, 25.7984) -> (-19.2358, 24.7984)
  line L6863 (-19.8454, 24.7984) -> (-20.8454, 24.7984)
  line L6864 (-20.8454, 24.7984) -> (-20.8454, 25.7984)
  line L6865 (-20.8454, 25.7984) -> (-19.8454, 25.7984)
  line L6866 (-19.8454, 25.7984) -> (-19.8454, 24.7984)
  line L6867 (-20.4677, 24.7984) -> (-21.4677, 24.7984)
  line L6868 (-21.4677, 24.7984) -> (-21.4677, 25.7984)
  line L6869 (-21.4677, 25.7984) -> (-20.4677, 25.7984)
  line L6870 (-20.4677, 25.7984) -> (-20.4677, 24.7984)
  line L6871 (-21.471, 24.7984) -> (-22.471, 24.7984)
  line L6872 (-22.471, 24.7984) -> (-22.471, 25.7984)
  line L6873 (-22.471, 25.7984) -> (-21.471, 25.7984)
  line L6874 (-21.471, 25.7984) -> (-21.471, 24.7984)
  line L6875 (-12.9874, 24.8238) -> (-13.9874, 24.8238)
  line L6876 (-13.9874, 24.8238) -> (-13.9874, 25.8238)
  line L6877 (-13.9874, 25.8238) -> (-12.9874, 25.8238)
  line L6878 (-12.9874, 25.8238) -> (-12.9874, 24.8238)
  line L6879 (-13.8002, 24.8238) -> (-14.8002, 24.8238)
  line L6880 (-14.8002, 24.8238) -> (-14.8002, 25.8238)
  line L6881 (-14.8002, 25.8238) -> (-13.8002, 25.8238)
  line L6882 (-13.8002, 25.8238) -> (-13.8002, 24.8238)
  line L6883 (-14.6638, 24.8238) -> (-15.6638, 24.8238)
  line L6884 (-15.6638, 24.8238) -> (-15.6638, 25.8238)
  line L6885 (-15.6638, 25.8238) -> (-14.6638, 25.8238)
  line L6886 (-14.6638, 25.8238) -> (-14.6638, 24.8238)
  line L6887 (-15.4766, 24.8238) -> (-16.4766, 24.8238)
  line L6888 (-16.4766, 24.8238) -> (-16.4766, 25.8238)
  line L6889 (-16.4766, 25.8238) -> (-15.4766, 25.8238)
  line L6890 (-15.4766, 25.8238) -> (-15.4766, 24.8238)
  line L6891 (-15.9846, 24.8238) -> (-16.9846, 24.8238)
  line L6892 (-16.9846, 24.8238) -> (-16.9846, 25.8238)
  line L6893 (-16.9846, 25.8238) -> (-15.9846, 25.8238)
  line L6894 (-15.9846, 25.8238) -> (-15.9846, 24.8238)
  line L6895 (-17.1022, 24.8238) -> (-18.1022, 24.8238)
  line L6896 (-18.1022, 24.8238) -> (-18.1022, 25.8238)
  line L6897 (-18.1022, 25.8238) -> (-17.1022, 25.8238)
  line L6898 (-17.1022, 25.8238) -> (-17.1022, 24.8238)
  line L6899 (-17.915, 24.8238) -> (-18.915, 24.8238)
  line L6900 (-18.915, 24.8238) -> (-18.915, 25.8238)
  line L6901 (-18.915, 25.8238) -> (-17.915, 25.8238)
  line L6902 (-17.915, 25.8238) -> (-17.915, 24.8238)
  line L6903 (-18.677, 24.8238) -> (-19.677, 24.8238)
  line L6904 (-19.677, 24.8238) -> (-19.677, 25.8238)
  line L6905 (-19.677, 25.8238) -> (-18.677, 25.8238)
  line L6906 (-18.677, 25.8238) -> (-18.677, 24.8238)
  line L6907 (-19.2358, 24.8238) -> (-20.2358, 24.8238)
  line L6908 (-20.2358, 24.8238) -> (-20.2358, 25.8238)
  line L6909 (-20.2358, 25.8238) -> (-19.2358, 25.8238)
  line L6910 (-19.2358, 25.8238) -> (-19.2358, 24.8238)
  line L6911 (-19.8454, 24.8238) -> (-20.8454, 24.8238)
  line L6912 (-20.8454, 24.8238) -> (-20.8454, 25.8238)
  line L6913 (-20.8454, 25.8238) -> (-19.8454, 25.8238)
  line L6914 (-19.8454, 25.8238) -> (-19.8454, 24.8238)
  line L6915 (-20.4804, 24.8238) -> (-21.4804, 24.8238)
  line L6916 (-21.4804, 24.8238) -> (-21.4804, 25.8238)
  line L6917 (-21.4804, 25.8238) -> (-20.4804, 25.8238)
  line L6918 (-20.4804, 25.8238) -> (-20.4804, 24.8238)
  line L6919 (-21.471, 24.8238) -> (-22.471, 24.8238)
  line L6920 (-22.471, 24.8238) -> (-22.471, 25.8238)
  line L6921 (-22.471, 25.8238) -> (-21.471, 25.8238)
  line L6922 (-21.471, 25.8238) -> (-21.471, 24.8238)
  line L6923 (-12.9747, 24.8492) -> (-13.9747, 24.8492)
  line L6924 (-13.9747, 24.8492) -> (-13.9747, 25.8492)
  line L6925 (-13.9747, 25.8492) -> (-12.9747, 25.8492)
  line L6926 (-12.9747, 25.8492) -> (-12.9747, 24.8492)
  line L6927 (-13.7748, 24.8492) -> (-14.7748, 24.8492)
  line L6928 (-14.7748, 24.8492) -> (-14.7748, 25.8492)
  line L6929 (-14.7748, 25.8492) -> (-13.7748, 25.8492)
  line L6930 (-13.7748, 25.8492) -> (-13.7748, 24.8492)
  line L6931 (-14.6384, 24.8492) -> (-15.6384, 24.8492)
  line L6932 (-15.6384, 24.8492) -> (-15.6384, 25.8492)
  line L6933 (-15.6384, 25.8492) -> (-14.6384, 25.8492)
  line L6934 (-14.6384, 25.8492) -> (-14.6384, 24.8492)
  line L6935 (-15.7941, 24.8492) -> (-16.7941, 24.8492)
  line L6936 (-16.7941, 24.8492) -> (-16.7941, 25.8492)
  line L6937 (-16.7941, 25.8492) -> (-15.7941, 25.8492)
  line L6938 (-15.7941, 25.8492) -> (-15.7941, 24.8492)
  line L6939 (-17.1022, 24.8492) -> (-18.1022, 24.8492)
  line L6940 (-18.1022, 24.8492) -> (-18.1022, 25.8492)
  line L6941 (-18.1022, 25.8492) -> (-17.1022, 25.8492)
  line L6942 (-17.1022, 25.8492) -> (-17.1022, 24.8492)
  line L6943 (-17.9277, 24.8492) -> (-18.9277, 24.8492)
  line L6944 (-18.9277, 24.8492) -> (-18.9277, 25.8492)
  line L6945 (-18.9277, 25.8492) -> (-17.9277, 25.8492)
  line L6946 (-17.9277, 25.8492) -> (-17.9277, 24.8492)
  line L6947 (-18.677, 24.8492) -> (-19.677, 24.8492)
  line L6948 (-19.677, 24.8492) -> (-19.677, 25.8492)
  line L6949 (-19.677, 25.8492) -> (-18.677, 25.8492)
  line L6950 (-18.677, 25.8492) -> (-18.677, 24.8492)
  line L6951 (-19.2358, 24.8492) -> (-20.2358, 24.8492)
  line L6952 (-20.2358, 24.8492) -> (-20.2358, 25.8492)
  line L6953 (-20.2358, 25.8492) -> (-19.2358, 25.8492)
  line L6954 (-19.2358, 25.8492) -> (-19.2358, 24.8492)
  line L6955 (-19.8454, 24.8492) -> (-20.8454, 24.8492)
  line L6956 (-20.8454, 24.8492) -> (-20.8454, 25.8492)
  line L6957 (-20.8454, 25.8492) -> (-19.8454, 25.8492)
  line L6958 (-19.8454, 25.8492) -> (-19.8454, 24.8492)
  line L6959 (-20.4804, 24.8492) -> (-21.4804, 24.8492)
  line L6960 (-21.4804, 24.8492) -> (-21.4804, 25.8492)
  line L6961 (-21.4804, 25.8492) -> (-20.4804, 25.8492)
  line L6962 (-20.4804, 25.8492) -> (-20.4804, 24.8492)
  line L6963 (-21.471, 24.8492) -> (-22.471, 24.8492)
  line L6964 (-22.471, 24.8492) -> (-22.471, 25.8492)
  line L6965 (-22.471, 25.8492) -> (-21.471, 25.8492)
  line L6966 (-21.471, 25.8492) -> (-21.471, 24.8492)
  line L6967 (-12.962, 24.8746) -> (-13.962, 24.8746)
  line L6968 (-13.962, 24.8746) -> (-13.962, 25.8746)
  line L6969 (-13.962, 25.8746) -> (-12.962, 25.8746)
  line L6970 (-12.962, 25.8746) -> (-12.962, 24.8746)
  line L6971 (-13.7494, 24.8746) -> (-14.7494, 24.8746)
  line L6972 (-14.7494, 24.8746) -> (-14.7494, 25.8746)
  line L6973 (-14.7494, 25.8746) -> (-13.7494, 25.8746)
  line L6974 (-13.7494, 25.8746) -> (-13.7494, 24.8746)
  line L6975 (-14.6257, 24.8746) -> (-15.6257, 24.8746)
  line L6976 (-15.6257, 24.8746) -> (-15.6257, 25.8746)
  line L6977 (-15.6257, 25.8746) -> (-14.6257, 25.8746)
  line L6978 (-14.6257, 25.8746) -> (-14.6257, 24.8746)
  line L6979 (-15.8068, 24.8746) -> (-16.8068, 24.8746)
  line L6980 (-16.8068, 24.8746) -> (-16.8068, 25.8746)
  line L6981 (-16.8068, 25.8746) -> (-15.8068, 25.8746)
  line L6982 (-15.8068, 25.8746) -> (-15.8068, 24.8746)
  line L6983 (-17.0895, 24.8746) -> (-18.0895, 24.8746)
  line L6984 (-18.0895, 24.8746) -> (-18.0895, 25.8746)
  line L6985 (-18.0895, 25.8746) -> (-17.0895, 25.8746)
  line L6986 (-17.0895, 25.8746) -> (-17.0895, 24.8746)
  line L6987 (-17.9404, 24.8746) -> (-18.9404, 24.8746)
  line L6988 (-18.9404, 24.8746) -> (-18.9404, 25.8746)
  line L6989 (-18.9404, 25.8746) -> (-17.9404, 25.8746)
  line L6990 (-17.9404, 25.8746) -> (-17.9404, 24.8746)
  line L6991 (-18.677, 24.8746) -> (-19.677, 24.8746)
  line L6992 (-19.677, 24.8746) -> (-19.677, 25.8746)
  line L6993 (-19.677, 25.8746) -> (-18.677, 25.8746)
  line L6994 (-18.677, 25.8746) -> (-18.677, 24.8746)
  line L6995 (-19.2358, 24.8746) -> (-20.2358, 24.8746)
  line L6996 (-20.2358, 24.8746) -> (-20.2358, 25.8746)
  line L6997 (-20.2358, 25.8746) -> (-19.2358, 25.8746)
  line L6998 (-19.2358, 25.8746) -> (-19.2358, 24.8746)
  line L6999 (-19.8581, 24.8746) -> (-20.8581, 24.8746)
  line L7000 (-20.8581, 24.8746) -> (-20.8581, 25.8746)
  line L7001 (-20.8581, 25.8746) -> (-19.8581, 25.8746)
  line L7002 (-19.8581, 25.8746) -> (-19.8581, 24.8746)
  line L7003 (-20.4804, 24.8746) -> (-21.4804, 24.8746)
  line L7004 (-21.4804, 24.8746) -> (-21.4804, 25.8746)
  line L7005 (-21.4804, 25.8746) -> (-20.4804, 25.8746)
  line L7006 (-20.4804, 25.8746) -> (-20.4804, 24.8746)
  line L7007 (-21.4837, 24.8746) -> (-22.4837, 24.8746)
  line L7008 (-22.4837, 24.8746) -> (-22.4837, 25.8746)
  line L7009 (-22.4837, 25.8746) -> (-21.4837, 25.8746)
  line L7010 (-21.4837, 25.8746) -> (-21.4837, 24.8746)
  line L7011 (-12.9493, 24.9) -> (-13.9493, 24.9)
  line L7012 (-13.9493, 24.9) -> (-13.9493, 25.9)
  line L7013 (-13.9493, 25.9) -> (-12.9493, 25.9)
  line L7014 (-12.9493, 25.9) -> (-12.9493, 24.9)
  line L7015 (-13.7367, 24.9) -> (-14.7367, 24.9)
  line L7016 (-14.7367, 24.9) -> (-14.7367, 25.9)
  line L7017 (-14.7367, 25.9) -> (-13.7367, 25.9)
  line L7018 (-13.7367, 25.9) -> (-13.7367, 24.9)
  line L7019 (-14.6257, 24.9) -> (-15.6257, 24.9)
  line L7020 (-15.6257, 24.9) -> (-15.6257, 25.9)
  line L7021 (-15.6257, 25.9) -> (-14.6257, 25.9)
  line L7022 (-14.6257, 25.9) -> (-14.6257, 24.9)
  line L7023 (-15.8195, 24.9) -> (-16.8195, 24.9)
  line L7024 (-16.8195, 24.9) -> (-16.8195, 25.9)
  line L7025 (-16.8195, 25.9) -> (-15.8195, 25.9)
  line L7026 (-15.8195, 25.9) -> (-15.8195, 24.9)
  line L7027 (-17.0768, 24.9) -> (-18.0768, 24.9)
  line L7028 (-18.0768, 24.9) -> (-18.0768, 25.9)
  line L7029 (-18.0768, 25.9) -> (-17.0768, 25.9)
  line L7030 (-17.0768, 25.9) -> (-17.0768, 24.9)
  line L7031 (-17.9404, 24.9) -> (-18.9404, 24.9)
  line L7032 (-18.9404, 24.9) -> (-18.9404, 25.9)
  line L7033 (-18.9404, 25.9) -> (-17.9404, 25.9)
  line L7034 (-17.9404, 25.9) -> (-17.9404, 24.9)
  line L7035 (-18.677, 24.9) -> (-19.677, 24.9)
  line L7036 (-19.677, 24.9) -> (-19.677, 25.9)
  line L7037 (-19.677, 25.9) -> (-18.677, 25.9)
  line L7038 (-18.677, 25.9) -> (-18.677, 24.9)
  line L7039 (-19.2358, 24.9) -> (-20.2358, 24.9)
  line L7040 (-20.2358, 24.9) -> (-20.2358, 25.9)
  line L7041 (-20.2358, 25.9) -> (-19.2358, 25.9)
  line L7042 (-19.2358, 25.9) -> (-19.2358, 24.9)
  line L7043 (-19.8454, 24.9) -> (-20.8454, 24.9)
  line L7044 (-20.8454, 24.9) -> (-20.8454, 25.9)
  line L7045 (-20.8454, 25.9) -> (-19.8454, 25.9)
  line L7046 (-19.8454, 25.9) -> (-19.8454, 24.9)
  line L7047 (-20.4804, 24.9) -> (-21.4804, 24.9)
  line L7048 (-21.4804, 24.9) -> (-21.4804, 25.9)
  line L7049 (-21.4804, 25.9) -> (-20.4804, 25.9)
  line L7050 (-20.4804, 25.9) -> (-20.4804, 24.9)
  line L7051 (-21.471, 24.9) -> (-22.471, 24.9)
  line L7052 (-22.471, 24.9) -> (-22.471, 25.9)
  line L7053 (-22.471, 25.9) -> (-21.471, 25.9)
  line L7054 (-21.471, 25.9) -> (-21.471, 24.9)
  line L7055 (-12.9493, 24.9254) -> (-13.9493, 24.9254)
  line L7056 (-13.9493, 24.9254) -> (-13.9493, 25.9254)
  line L7057 (-13.9493, 25.9254) -> (-12.9493, 25.9254)
  line L7058 (-12.9493, 25.9254) -> (-12.9493, 24.9254)
  line L7059 (-13.7113, 24.9254) -> (-14.7113, 24.9254)
  line L7060 (-14.7113, 24.9254) -> (-14.7113, 25.9254)
  line L7061 (-14.7113, 25.9254) -> (-13.7113, 25.9254)
  line L7062 (-13.7113, 25.9254) -> (-13.7113, 24.9254)
  line L7063 (-14.6003, 24.9254) -> (-15.6003, 24.9254)
  line L7064 (-15.6003, 24.9254) -> (-15.6003, 25.9254)
  line L7065 (-15.6003, 25.9254) -> (-14.6003, 25.9254)
  line L7066 (-14.6003, 25.9254) -> (-14.6003, 24.9254)
  line L7067 (-15.8322, 24.9254) -> (-16.8322, 24.9254)
  line L7068 (-16.8322, 24.9254) -> (-16.8322, 25.9254)
  line L7069 (-16.8322, 25.9254) -> (-15.8322, 25.9254)
  line L7070 (-15.8322, 25.9254) -> (-15.8322, 24.9254)
  line L7071 (-17.0641, 24.9254) -> (-18.0641, 24.9254)
  line L7072 (-18.0641, 24.9254) -> (-18.0641, 25.9254)
  line L7073 (-18.0641, 25.9254) -> (-17.0641, 25.9254)
  line L7074 (-17.0641, 25.9254) -> (-17.0641, 24.9254)
  line L7075 (-17.9404, 24.9254) -> (-18.9404, 24.9254)
  line L7076 (-18.9404, 24.9254) -> (-18.9404, 25.9254)
  line L7077 (-18.9404, 25.9254) -> (-17.9404, 25.9254)
  line L7078 (-17.9404, 25.9254) -> (-17.9404, 24.9254)
  line L7079 (-18.677, 24.9254) -> (-19.677, 24.9254)
  line L7080 (-19.677, 24.9254) -> (-19.677, 25.9254)
  line L7081 (-19.677, 25.9254) -> (-18.677, 25.9254)
  line L7082 (-18.677, 25.9254) -> (-18.677, 24.9254)
  line L7083 (-19.2358, 24.9254) -> (-20.2358, 24.9254)
  line L7084 (-20.2358, 24.9254) -> (-20.2358, 25.9254)
  line L7085 (-20.2358, 25.9254) -> (-19.2358, 25.9254)
  line L7086 (-19.2358, 25.9254) -> (-19.2358, 24.9254)
  line L7087 (-19.8454, 24.9254) -> (-20.8454, 24.9254)
  line L7088 (-20.8454, 24.9254) -> (-20.8454, 25.9254)
  line L7089 (-20.8454, 25.9254) -> (-19.8454, 25.9254)
  line L7090 (-19.8454, 25.9254) -> (-19.8454, 24.9254)
  line L7091 (-20.4804, 24.9254) -> (-21.4804, 24.9254)
  line L7092 (-21.4804, 24.9254) -> (-21.4804, 25.9254)
  line L7093 (-21.4804, 25.9254) -> (-20.4804, 25.9254)
  line L7094 (-20.4804, 25.9254) -> (-20.4804, 24.9254)
  line L7095 (-21.4837, 24.9254) -> (-22.4837, 24.9254)
  line L7096 (-22.4837, 24.9254) -> (-22.4837, 25.9254)
  line L7097 (-22.4837, 25.9254) -> (-21.4837, 25.9254)
  line L7098 (-21.4837, 25.9254) -> (-21.4837, 24.9254)
  line L7099 (-12.9366, 24.9508) -> (-13.9366, 24.9508)
  line L7100 (-13.9366, 24.9508) -> (-13.9366, 25.9508)
  line L7101 (-13.9366, 25.9508) -> (-12.9366, 25.9508)
  line L7102 (-12.9366, 25.9508) -> (-12.9366, 24.9508)
  line L7103 (-13.6859, 24.9508) -> (-14.6859, 24.9508)
  line L7104 (-14.6859, 24.9508) -> (-14.6859, 25.9508)
  line L7105 (-14.6859, 25.9508) -> (-13.6859, 25.9508)
  line L7106 (-13.6859, 25.9508) -> (-13.6859, 24.9508)
  line L7107 (-14.5876, 24.9508) -> (-15.5876, 24.9508)
  line L7108 (-15.5876, 24.9508) -> (-15.5876, 25.9508)
  line L7109 (-15.5876, 25.9508) -> (-14.5876, 25.9508)
  line L7110 (-14.5876, 25.9508) -> (-14.5876, 24.9508)
  line L7111 (-15.8322, 24.9508) -> (-16.8322, 24.9508)
  line L7112 (-16.8322, 24.9508) -> (-16.8322, 25.9508)
  line L7113 (-16.8322, 25.9508) -> (-15.8322, 25.9508)
  line L7114 (-15.8322, 25.9508) -> (-15.8322, 24.9508)
  line L7115 (-17.0514, 24.9508) -> (-18.0514, 24.9508)
  line L7116 (-18.0514, 24.9508) -> (-18.0514, 25.9508)
  line L7117 (-18.0514, 25.9508) -> (-17.0514, 25.9508)
  line L7118 (-17.0514, 25.9508) -> (-17.0514, 24.9508)
  line L7119 (-17.9404, 24.9508) -> (-18.9404, 24.9508)
  line L7120 (-18.9404, 24.9508) -> (-18.9404, 25.9508)
  line L7121 (-18.9404, 25.9508) -> (-17.9404, 25.9508)
  line L7122 (-17.9404, 25.9508) -> (-17.9404, 24.9508)
  line L7123 (-18.677, 24.9508) -> (-19.677, 24.9508)
  line L7124 (-19.677, 24.9508) -> (-19.677, 25.9508)
  line L7125 (-19.677, 25.9508) -> (-18.677, 25.9508)
  line L7126 (-18.677, 25.9508) -> (-18.677, 24.9508)
  line L7127 (-19.2358, 24.9508) -> (-20.2358, 24.9508)
  line L7128 (-20.2358, 24.9508) -> (-20.2358, 25.9508)
  line L7129 (-20.2358, 25.9508) -> (-19.2358, 25.9508)
  line L7130 (-19.2358, 25.9508) -> (-19.2358, 24.9508)
  line L7131 (-19.8581, 24.9508) -> (-20.8581, 24.9508)
  line L7132 (-20.8581, 24.9508) -> (-20.8581, 25.9508)
  line L7133 (-20.8581, 25.9508) -> (-19.8581, 25.9508)
  line L7134 (-19.8581, 25.9508) -> (-19.8581, 24.9508)
  line L7135 (-20.4804, 24.9508) -> (-21.4804, 24.9508)
  line L7136 (-21.4804, 24.9508) -> (-21.4804, 25.9508)
  line L7137 (-21.4804, 25.9508) -> (-20.4804, 25.9508)
  line L7138 (-20.4804, 25.9508) -> (-20.4804, 24.9508)
  line L7139 (-21.4837, 24.9508) -> (-22.4837, 24.9508)
  line L7140 (-22.4837, 24.9508) -> (-22.4837, 25.9508)
  line L7141 (-22.4837, 25.9508) -> (-21.4837, 25.9508)
  line L7142 (-21.4837, 25.9508) -> (-21.4837, 24.9508)
  line L7143 (-12.9366, 24.9762) -> (-13.9366, 24.9762)
  line L7144 (-13.9366, 24.9762) -> (-13.9366, 25.9762)
  line L7145 (-13.9366, 25.9762) -> (-12.9366, 25.9762)
  line L7146 (-12.9366, 25.9762) -> (-12.9366, 24.9762)
  line L7147 (-13.6732, 24.9762) -> (-14.6732, 24.9762)
  line L7148 (-14.6732, 24.9762) -> (-14.6732, 25.9762)
  line L7149 (-14.6732, 25.9762) -> (-13.6732, 25.9762)
  line L7150 (-13.6732, 25.9762) -> (-13.6732, 24.9762)
  line L7151 (-14.5749, 24.9762) -> (-15.5749, 24.9762)
  line L7152 (-15.5749, 24.9762) -> (-15.5749, 25.9762)
  line L7153 (-15.5749, 25.9762) -> (-14.5749, 25.9762)
  line L7154 (-14.5749, 25.9762) -> (-14.5749, 24.9762)
  line L7155 (-15.8449, 24.9762) -> (-16.8449, 24.9762)
  line L7156 (-16.8449, 24.9762) -> (-16.8449, 25.9762)
  line L7157 (-16.8449, 25.9762) -> (-15.8449, 25.9762)
  line L7158 (-15.8449, 25.9762) -> (-15.8449, 24.9762)
  line L7159 (-17.0514, 24.9762) -> (-18.0514, 24.9762)
  line L7160 (-18.0514, 24.9762) -> (-18.0514, 25.9762)
  line L7161 (-18.0514, 25.9762) -> (-17.0514, 25.9762)
  line L7162 (-17.0514, 25.9762) -> (-17.0514, 24.9762)
  line L7163 (-17.9404, 24.9762) -> (-18.9404, 24.9762)
  line L7164 (-18.9404, 24.9762) -> (-18.9404, 25.9762)
  line L7165 (-18.9404, 25.9762) -> (-17.9404, 25.9762)
  line L7166 (-17.9404, 25.9762) -> (-17.9404, 24.9762)
  line L7167 (-18.677, 24.9762) -> (-19.677, 24.9762)
  line L7168 (-19.677, 24.9762) -> (-19.677, 25.9762)
  line L7169 (-19.677, 25.9762) -> (-18.677, 25.9762)
  line L7170 (-18.677, 25.9762) -> (-18.677, 24.9762)
  line L7171 (-19.2358, 24.9762) -> (-20.2358, 24.9762)
  line L7172 (-20.2358, 24.9762) -> (-20.2358, 25.9762)
  line L7173 (-20.2358, 25.9762) -> (-19.2358, 25.9762)